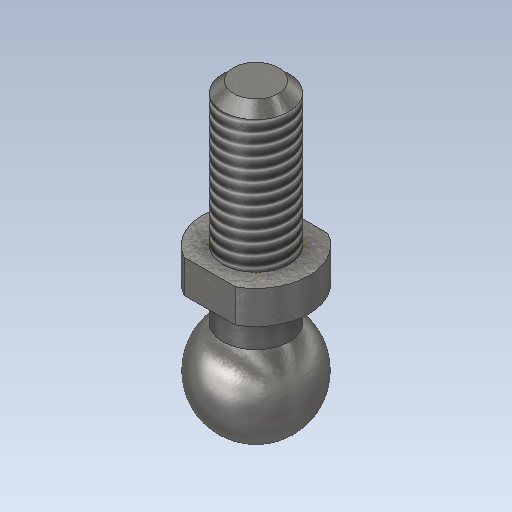
# Autodesk Inventor part: Ball_Joint_Ball
Saved by Autodesk Inventor 2021.4 (Build 254397000, 397)
## iProperties
Created: 2020-05-14
Part Number: Ball_Joint_Ball
Material: Stahl, galvanisiert
Document SubType Name: Modeling
Designer: Alex
Density: 7.85 g/cm^3
Appearance: Galvanisiert
Mass: 4.99585 g
Surface Area: 5.18593 cm^2
Volume: 0.636414 cm^3
Author: Alex
Autodesk Inventor part; units mm, degrees
ref_plane "YZ Plane" through (0, 0, 0) normal (1, 0, 0) x (0, 1, 0)
ref_plane "XY Plane" through (0, 0, 0) normal (0, 0, 1) x (1, 0, 0)
sketch "Skizze1" plane through (0, 0, 0) normal (0, 0, 1) x (1, 0, 0)
  arc A0 (0, 4) -> (0, -4) centre (0, 0) ccw
  line L0 (0, 4) -> (0, -4)
  line L1 (0, -5.6) -> (0, 5.6) construction
  dimension "d0" = 8
  constraints: 2 coincident, 2 end point, 2 point on circle, 1 centre point, 1 collinear, 1 vertical
  measures "d0" diameter of A0
revolve "Kugelkörper" add sketch "Skizze1" angle 360 about axis through (0, -10, 0) along (0, 1, 0)
ref_plane "Konstruktionshilfsebene" through (0, 4, 0) normal (0, 1, 0) x (-1, 0, 0)
sketch "Skizze2" plane through (0, 4, 0) normal (0, 1, 0) x (-1, 0, 0)
  circle A0 centre (0, 0) radius 2.5
  point P0 (0, 0)
  dimension "d2" = 5
  constraints: 1 centre point, 1 coincident
  measures "d2" diameter of A0
extrude "Gewindeschraube" add sketch "Skizze2" against normal blind 1 and the other way blind 15
chamfer "Gewindefase M3" distance 0.8 angle 45 1 edges at (2.5, 19, 0)
ref_plane "Work Plane2" through (0, 8.2, 0) normal (0, 1, 0) x (1, 0, 0)
sketch "Sketch3" plane through (0, 8.2, 0) normal (0, 1, 0) x (1, 0, 0)
  circle A0 centre (0, 0) radius 4
  line L0 (-1.9365, -3.5) -> (1.9365, -3.5)
  line L1 (-1.9365, 3.5) -> (1.9365, 3.5)
  dimension "d13" = 8
  dimension "d14" = 7
  constraints: 4 end point, 4 point on circle, 2 parallel, 1 centre point, 1 coincident, 1 horizontal
  measures "d13" diameter of A0
  measures "d14" distance between parallel lines of L1 L0
extrude "Extrusion2" add sketch "Sketch3" against normal blind 2.5 contours A0 L0 L1
thread "Thread2" size "M5x0.8" class "6g" standard "ANSI Metric M Profile" full length
